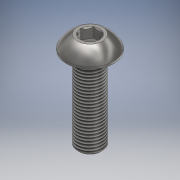
# Autodesk Inventor part: Bolt_M3x0.35_10mm_BH
Saved by Autodesk Inventor 2018 (Build 220112000, 112)
## iProperties
Created: 2017-10-22
Part Number: Bolt_M3x0.35_10mm_BH
Material: Stainless Steel
Document SubType Name: Modeling
Designer: Bradley
Density: 8 g/cm^3
Appearance: Semi-Polished
Author: Bradley
Autodesk Inventor part; units mm, degrees
ref_plane "YZ Plane" through (0, 0, 0) normal (1, 0, 0) x (0, 1, 0)
ref_plane "XZ Plane" through (0, 0, 0) normal (0, 1, 0) x (-1, 0, 0)
ref_plane "XY Plane" through (0, 0, 0) normal (0, 0, 1) x (1, 0, 0)
sketch "Sketch1" plane through (0, 0, 0) normal (0, 1, 0) x (-1, 0, 0)
  line L0 (0, 5.2476) -> (0, -5.2476)
  line L1 (0, -5.2476) -> (-1.25, -5.2476)
  line L2 (-1.25, -5.2476) -> (-1.5, -4.9976)
  line L3 (-1.5, -4.9976) -> (-1.5, 4.6524)
  line L4 (-1.6, 4.7524) -> (-2.85, 4.7524)
  line L5 (-2.85, 4.7524) -> (-2.85, 5.0024)
  line L6 (0, 5.2476) -> (-1.1547, 6.4024)
  line L7 (-1.1547, 6.4024) -> (-1.5, 6.4024)
  arc A0 (-1.5, 6.4024) -> (-2.85, 5.0024) centre (0, 3.605) ccw
  line L8 (-1.1547, 6.4024) -> (-0.5774, 7.4024) construction
  line L9 (-0.5774, 7.4024) -> (0.5774, 7.4024) construction
  line L10 (0.5774, 7.4024) -> (1.1547, 6.4024) construction
  line L11 (1.1547, 6.4024) -> (0.5774, 5.4024) construction
  line L12 (0.5774, 5.4024) -> (-0.5774, 5.4024) construction
  line L13 (-0.5774, 5.4024) -> (-1.1547, 6.4024) construction
  arc A1 (-1.5, 4.6524) -> (-1.6, 4.7524) centre (-1.6, 4.6524) ccw
  point P0 (0, 0)
  point P1 (-1.5, 4.7524)
  point P2 (0, 0)
  point P3 (0, 6.4024)
  dimension "d0" = 3
  dimension "d1" = 10
  dimension "d2" = 0.25
  dimension "d3" = 135
  dimension "d4" = 5.7
  dimension "d5" = 3
  dimension "d6" = 1.65
  dimension "d7" = 2
  dimension "d8" = 0.25
  dimension "d15" = 3.2
  constraints: 28 end point, 4 point on circle, 4 point on line, 3 perpendicular, 2 centre point, 2 horizontal, 2 parallel, 2 tangent, 1 coincident, 1 midpoint, 1 vertical, 13 other
  measures "d0" diameter of L3 L0
  measures "d1" distance between parallel lines of L1 L4
  measures "d2" horizontal distance of L1.end L2.end
  measures "d3" angle of L3 L2
  measures "d4" diameter of L5 L0
  measures "d5" diameter of L7.end L0
  measures "d6" distance between parallel lines of L4 L7
  measures "d7" distance between parallel lines of L9 L12
  measures "d8" distance of L4.end L5.end
  measures "d15" diameter of L4.start L0
revolve "Revolution1" add sketch "Sketch1" angle 360 about axis through (0, 0, 5.2476) along (0, 0, -1)
sketch "Sketch2" plane through (0, 0, 6.4024) normal (0, 0, 1) x (1, 0, 0)
  circle A0 centre (0, 0) radius 1.1547 projected
  circle A1 centre (0, 0) radius 1.5 projected
  line L0 (-1.1547, 0) -> (-0.5774, 1)
  line L1 (-0.5774, 1) -> (0.5774, 1)
  line L2 (0.5774, 1) -> (1.1547, 0)
  line L3 (1.1547, 0) -> (0.5774, -1)
  line L4 (0.5774, -1) -> (-0.5774, -1)
  line L5 (-0.5774, -1) -> (-1.1547, 0)
  point P0 (0, 0)
  constraints: 12 end point, 1 coincident, 1 horizontal, 1 horizontal alignment, 14 other
extrude "Extrusion1" cut sketch "Sketch2" against normal blind 1.2 contours L3 L4 L5 L0 L1 L2
thread "Thread1" size "M3x0.35" class "6g" standard "ANSI Metric M Profile" full length
body "Solid1"
